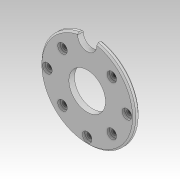
# Autodesk Inventor part: WristMotorPlate
Saved by Autodesk Inventor 2020 (Build 240168000, 168)
## iProperties
Created: 2022-04-02
Part Number: WristMotorPlate
Material: Generic
Document SubType Name: Modeling
Designer: DDeGo
Density: 1 g/cm^3
Appearance: Default
Author: DDeGo
Autodesk Inventor part; units mm, degrees
ref_plane "YZ Plane" through (0, 0, 0) normal (1, 0, 0) x (0, 1, 0)
ref_plane "XZ Plane" through (0, 0, 0) normal (0, 1, 0) x (-1, 0, 0)
ref_plane "XY Plane" through (0, 0, 0) normal (0, 0, 1) x (1, 0, 0)
sketch "Sketch1" plane through (0, 0, 0) normal (0, 0, 1) x (1, 0, 0)
  circle A0 centre (0, 0) radius 29.5
  line L0 (-15.5, -15.5) -> (15.5, -15.5) construction
  line L1 (15.5, -15.5) -> (15.5, 15.5) construction
  line L2 (15.5, 15.5) -> (-15.5, 15.5) construction
  line L3 (-15.5, 15.5) -> (-15.5, -15.5) construction
  line L4 (-15.5, -15.5) -> (15.5, 15.5) construction
  line L5 (15.5, -15.5) -> (-15.5, 15.5) construction
  circle A1 centre (-15.5, 15.5) radius 1.65
  circle A2 centre (15.5, 15.5) radius 1.65
  circle A3 centre (15.5, -15.5) radius 1.65
  circle A4 centre (-15.5, -15.5) radius 1.65
  circle A5 centre (0, 0) radius 11.5
  line L6 (0, 0) -> (25, 0) construction
  circle A6 centre (0, 0) radius 25 construction
  circle A7 centre (25, 0) radius 1.65
  circle A8 centre (-25, 0) radius 1.65
  circle A9 centre (0, -25) radius 1.65
  line L7 (-25, 0) -> (0, 0) construction
  line L8 (0, 0) -> (0, -25) construction
  dimension "d0" = 59
  dimension "d1" = 3.3
  dimension "d2" = 23
  dimension "d3" = 31
  dimension "d4" = 50
  dimension "d5" = 3.3
  constraints: 18 end point, 10 centre point, 8 coincident, 5 equal radius, 3 horizontal, 3 perpendicular, 3 point on circle, 2 midpoint, 2 parallel
  measures "d0" diameter of A0
  measures "d1" diameter of A1
  measures "d2" diameter of A5
  measures "d3" distance of L1.end L2.end
  measures "d4" diameter of A6
  measures "d5" diameter of A8
extrude "Extrusion1" add sketch "Sketch1" along normal blind 3.5
sketch "Sketch2" plane through (0, 0, 3.5) normal (0, 0, 1) x (1, 0, 0)
  circle A0 centre (0, -25) radius 1.65 projected
  circle A1 centre (0, -25) radius 3
  circle A2 centre (25, 0) radius 1.65 projected
  circle A3 centre (25, 0) radius 3
  circle A4 centre (-25, 0) radius 1.65 projected
  circle A5 centre (-25, 0) radius 3
  circle A6 centre (-15.5, -15.5) radius 1.65 projected
  circle A7 centre (-15.5, -15.5) radius 3
  circle A8 centre (15.5, -15.5) radius 1.65 projected
  circle A9 centre (15.5, -15.5) radius 3
  circle A10 centre (15.5, 15.5) radius 1.65 projected
  circle A11 centre (15.5, 15.5) radius 3
  circle A12 centre (-15.5, 15.5) radius 1.65 projected
  circle A13 centre (-15.5, 15.5) radius 3
  point P0 (0, 0)
  dimension "d8" = 6
  constraints: 7 centre point, 7 coincident, 6 equal radius
  measures "d8" diameter of A5
extrude "Extrusion2" cut sketch "Sketch2" against normal blind 1.5 contours A0 | A1 | A2 | A3 | A4 | A5 | A6 | A7 | A8 | A9 | A10 | A11 | A12 | A13
sketch "Sketch3" plane through (0, 0, 3.5) normal (0, 0, 1) x (1, 0, 0)
  line L0 (0, 31.5) -> (0, 27.5) construction
  circle A0 centre (0, 0) radius 29.5 construction
  line L1 (-6, 31.5) -> (-6, 27.5)
  line L2 (6, 27.5) -> (6, 31.5)
  arc A1 (6, 31.5) -> (-6, 31.5) centre (0, 31.5) ccw
  arc A2 (-6, 27.5) -> (6, 27.5) centre (0, 27.5) ccw
  point P0 (0, 29.5)
  dimension "d14" = 2
  dimension "d15" = 6
  constraints: 8 end point, 4 point on circle, 4 tangent, 2 centre point, 1 midpoint, 1 parallel, 1 point on line, 1 vertical, 1 vertical alignment, 1 other
  measures "d14" distance of L0.end point (0, 29.5)
  measures "d15" radius of A2
extrude "Extrusion3" cut sketch "Sketch3" against normal through all
chamfer "Chamfer1" distance 1 angle 45 2 edges at (0, -29.5, 3.5) (0, -29.5, 0)
body "Solid1"
